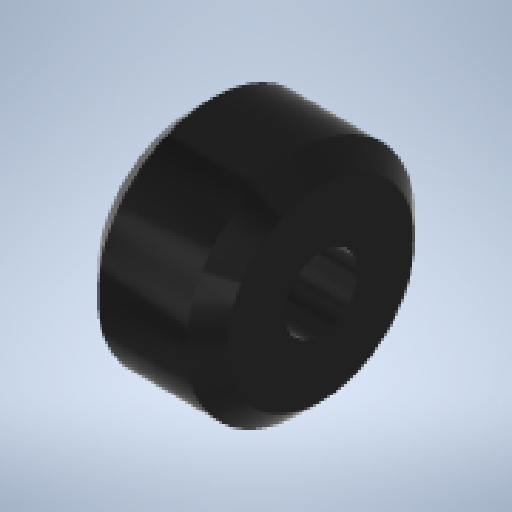
# Autodesk Inventor part: VSlotWheel
Saved by Autodesk Inventor 2023 (Build 270158000, 158)
## iProperties
Created: 2023-08-12
Part Number: VSlotWheel
Material: ABS Plastic
Document SubType Name: Modeling
Designer: Felix
Density: 1.06 g/cm^3
Appearance: Smooth - Black
Author: Felix
Autodesk Inventor part; units mm, degrees
ref_plane "YZ Plane" through (0, 0, 0) normal (1, 0, 0) x (0, 1, 0)
ref_plane "XZ Plane" through (0, 0, 0) normal (0, 1, 0) x (-1, 0, 0)
ref_plane "XY Plane" through (0, 0, 0) normal (0, 0, 1) x (1, 0, 0)
sketch "Sketch1" plane through (0, 0, 0) normal (0, 1, 0) x (-1, 0, 0)
  line L0 (0, 0) -> (8.8, 0)
  line L1 (8.8, 0) -> (8.8, -6.35)
  line L2 (7.4, -7.75) -> (1.4, -7.75)
  line L3 (0, -6.35) -> (0, 0)
  line L4 (7.4, -7.75) -> (8.8, -6.35)
  line L5 (1.4, -7.75) -> (0, -6.35)
  point P0 (8.8, -7.75)
  point P1 (0, -7.75)
  dimension "d0" = 7.75
  dimension "d1" = 8.8
  dimension "d6" = 6
  dimension "d7" = 1.4
  dimension "d8" = 1.4
  dimension "d9" = 135
  dimension "d10" = 135
  constraints: 12 end point, 4 point on line, 2 parallel, 1 horizontal, 1 perpendicular
  measures "d0" distance between parallel lines of L0 L2
  measures "d1" distance of point (8.8, -7.75) point (0, -7.75)
  measures "d6" distance of L2.start L2.end
  measures "d7" distance from line of L2.start L1
  measures "d8" horizontal distance of L2.end L3.start
  measures "d9" angle of L1 L4
  measures "d10" angle of L3 L5
revolve "Revolution1" add sketch "Sketch1" angle 360 about axis through (0, 0, 0) along (-1, 0, 0)
sketch "Sketch2" plane through (0, 0, 0) normal (1, 0, 0) x (0, 0, -1)
  circle A0 centre (0, 0) radius 6.35 construction
  circle A1 centre (0, 0) radius 2.45
  dimension "d12" = 4.9
  constraints: 1 centre point, 1 coincident
  measures "d12" diameter of A1
extrude "Extrusion1" cut sketch "Sketch2" against normal through all
equation "\"d8\" = d7"
equation "\"d10\" = d9"
body "Solid1"
